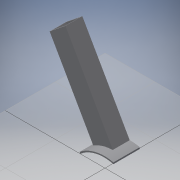
# Autodesk Inventor part: желоб
Saved by Autodesk Inventor 2019 (Build 230136000, 136)
## iProperties
Created: 2022-06-29
Part Number: желоб
Material: Типовые
Document SubType Name: Modeling
Designer: korsh
Density: 1 g/cm^3
Appearance: По умолчанию
Author: korsh
Autodesk Inventor part; units mm, degrees
ref_plane "YZ Plane" through (0, 0, 0) normal (1, 0, 0) x (0, 1, 0)
ref_plane "XZ Plane" through (0, 0, 0) normal (0, 1, 0) x (-1, 0, 0)
ref_plane "XY Plane" through (0, 0, 0) normal (0, 0, 1) x (1, 0, 0)
sketch "Эскиз1" plane through (0, 0, 0) normal (0, 0, 1) x (1, 0, 0)
  arc A0 (16.8748, 70) -> (-20.8748, 70) centre (-2, 0.0001) ccw projected
  arc A1 (-20.8748, 70) -> (-20.8744, -70) centre (-2, 0.0001) ccw projected
  line L0 (-41.3067, 60.92) -> (-46.4476, 70) projected
  arc A2 (16.8748, 70) -> (-49.6039, 54.682) centre (-2, 0.0001) ccw
  line L1 (16.8748, 70) -> (16.8748, 73)
  line L2 (-49.6039, 54.682) -> (-51.082, 57.2926)
  arc A3 (16.8748, 73) -> (-51.082, 57.2926) centre (-1.1236, -3.9899) ccw
  point P0 (0, 0)
  dimension "d0" = 3
  dimension "d1" = 3
  constraints: 6 point on circle, 4 end point, 2 centre point, 1 concentric, 1 vertical
  measures "d0" distance of L1.start L1.end
  measures "d1" distance of L2.start L2.end
extrude "Выдавливание1" add sketch "Эскиз1" against normal blind 19
sketch "Эскиз3" plane through (0, 0, -19) normal (0, 0, -1) x (-1, 0, 0)
  line L0 (-16.8748, 73) -> (-16.8748, 70) projected
  arc A0 (49.6039, 54.682) -> (-16.8748, 70) centre (2, 0.0001) ccw projected
  line L1 (49.6039, 54.682) -> (51.082, 57.2926) projected
  arc A1 (51.082, 57.2926) -> (-16.8748, 73) centre (1.1236, -3.9899) ccw projected
  line L2 (46.4476, 70) -> (41.3067, 60.92) projected
  line L3 (43.8771, 65.46) -> (130.1352, 217.8105)
  line L4 (2, 72.5001) -> (98.5921, 243.1026)
  line L5 (98.5921, 243.1026) -> (130.1352, 217.8105)
  arc A2 (51.082, 57.2926) -> (-16.8748, 73) centre (1.1236, -3.9899) ccw projected
  arc A3 (51.082, 57.2926) -> (42.65, 63.2927) centre (1.1236, -3.9899) ccw
  arc A4 (49.6039, 54.682) -> (-16.8748, 70) centre (2, 0.0001) ccw projected
  arc A5 (49.6039, 54.682) -> (41.3067, 60.92) centre (2, 0.0001) ccw
  line L6 (41.3067, 60.92) -> (42.65, 63.2927)
  line L7 (49.6039, 54.682) -> (51.082, 57.2926) projected
  line L8 (49.6039, 54.682) -> (51.082, 57.2926)
  arc A6 (3.4391, 75.0419) -> (-16.8748, 73) centre (1.1236, -3.9899) ccw
  line L9 (-16.8748, 73) -> (-16.8748, 70) projected
  arc A7 (2, 72.5001) -> (-16.8748, 70) centre (2, 0.0001) ccw
  line L10 (-16.8748, 73) -> (-16.8748, 70)
  line L11 (2, 72.5001) -> (3.4391, 75.0419)
  point P0 (0, 0)
  point P1 (0.1112, 66.9734)
  dimension "d8" = 180
  constraints: 14 end point, 10 point on circle, 4 centre point, 3 collinear, 2 concentric, 2 point on line, 1 midpoint, 2 other
  measures "d8" angle of L2 L3
extrude "Выдавливание2" add sketch "Эскиз3" along normal blind 3
sketch "Эскиз4" plane through (0, 0, -22) normal (0, 0, -1) x (-1, 0, 0)
  line L0 (49.6039, 54.682) -> (51.082, 57.2926) projected
  arc A0 (51.082, 57.2926) -> (42.65, 63.2927) centre (1.1236, -3.9899) ccw projected
  line L1 (42.65, 63.2927) -> (130.1352, 217.8105) projected
  line L2 (130.1352, 217.8105) -> (98.5921, 243.1026) projected
  line L3 (98.5921, 243.1026) -> (3.4391, 75.0419) projected
  arc A1 (3.4391, 75.0419) -> (-16.8748, 73) centre (1.1236, -3.9899) ccw projected
  line L4 (-16.8748, 73) -> (-16.8748, 70) projected
  arc A2 (49.6039, 54.682) -> (-16.8748, 70) centre (2, 0.0001) ccw projected
  line L5 (130.1352, 217.8105) -> (98.5921, 243.1026) projected
  line L6 (100.9326, 241.2259) -> (5.4025, 72.4202)
  arc A3 (49.6039, 54.682) -> (-16.8748, 70) centre (2, 0.0001) ccw projected
  line L7 (127.7947, 219.6872) -> (38.8155, 62.457)
  point P0 (0, 0)
  dimension "d14" = 3
  dimension "d15" = 3
  dimension "d16" = 3
  constraints: 4 end point, 2 point on circle, 2 point on line, 1 parallel
  measures "d14" distance of L2.end L6.start
  measures "d15" distance from line of L3.end L6
  measures "d16" distance of L1.end L7.start
extrude "Выдавливание3" add sketch "Эскиз4" along normal blind 28 contours A2 L7 L2 L1 A0 L0 | A2 L4 A1 L3 L2 L6
sketch "Эскиз5" plane through (0, 0, -50) normal (0, 0, -1) x (-1, 0, 0)
  line L0 (98.5921, 243.1026) -> (3.4391, 75.0419) projected
  arc A0 (3.4391, 75.0419) -> (-16.8748, 73) centre (1.1236, -3.9899) ccw projected
  arc A1 (5.4025, 72.4202) -> (-16.8748, 70) centre (2, 0.0001) ccw projected
  arc A2 (38.8155, 62.457) -> (5.4025, 72.4202) centre (2, 0.0001) ccw projected
  arc A3 (49.6039, 54.682) -> (38.8155, 62.457) centre (2, 0.0001) ccw projected
  arc A4 (51.082, 57.2926) -> (42.65, 63.2927) centre (1.1236, -3.9899) ccw projected
  line L1 (49.6039, 54.682) -> (51.082, 57.2926) projected
  line L2 (-16.8748, 73) -> (-16.8748, 70) projected
  line L3 (42.65, 63.2927) -> (130.1352, 217.8105) projected
  line L4 (98.5921, 243.1026) -> (130.1352, 217.8105)
  point P0 (0, 0)
  constraints: 2 end point
extrude "Выдавливание4" add sketch "Эскиз5" along normal blind 3
